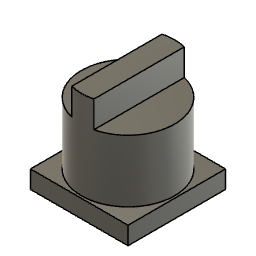
switch_knob (Autodesk Fusion 360 design; units mm, degrees)
Autodesk Fusion 360 part; units mm, degrees
sketch "Sketch1" plane through (0, 0, 0) normal (0, 1, 0) x (1, 0, 0)
  line L0 (5.5, 5.5) -> (-5.5, 5.5)
  line L1 (-5.5, 5.5) -> (-5.5, -5.5)
  line L2 (-5.5, -5.5) -> (5.5, -5.5)
  line L3 (5.5, -5.5) -> (5.5, 5.5)
  line L4 (5.5, 5.5) -> (-5.5, -5.5) construction
  line L5 (-5.5, 5.5) -> (5.5, -5.5) construction
  dimension "d1" = 11
  dimension "d2" = 11
  constraint horizontal L0
  constraint perpendicular L0 L1
  constraint parallel L0 L2
  constraint parallel L1 L3
  constraint coincident L4 origin
  constraint coincident L5 origin
  measures "d1" distance of L1.end L2.end
  measures "d2" distance of L0.end L1.end
extrude "Extrude1" add sketch "Sketch1" along normal blind 2
sketch "Sketch2" plane through (0, 2, 0) normal (0, 1, 0) x (-1, 0, 0)
  line L0 (-5.5, 5.5) -> (-5.5, -5.5)
  line L1 (-5.5, -5.5) -> (5.5, -5.5)
  line L2 (5.5, -5.5) -> (5.5, 5.5)
  line L3 (5.5, 5.5) -> (-5.5, 5.5)
  circle A0 centre (0, 0) radius 5.25
  dimension "d5" = 10.5
  constraint coincident A0.centre origin
  measures "d5" diameter of A0
extrude "Extrude2" add sketch "Sketch2" along normal blind 7 contours A0
sketch "Sketch3" plane through (0, 9, 0) normal (0, 1, 0) x (-1, 0, 0)
  circle A0 centre (0, 0) radius 5.25
  line L0 (1.25, 5.25) -> (-1.25, 5.25)
  line L1 (-1.25, 5.25) -> (-1.25, -5.25)
  line L2 (-1.25, -5.25) -> (1.25, -5.25)
  line L3 (1.25, -5.25) -> (1.25, 5.25)
  line L4 (1.25, 5.25) -> (-1.25, -5.25) construction
  line L5 (-1.25, 5.25) -> (1.25, -5.25) construction
  dimension "d8" = 2.5
  dimension "d9" = 10.5
  constraint horizontal L0
  constraint perpendicular L0 L1
  constraint parallel L0 L2
  constraint parallel L1 L3
  constraint coincident L4 A0.centre
  constraint coincident L5 A0.centre
  constraint coincident A0.centre origin
  measures "d8" distance of L1.end L2.end
  measures "d9" distance of L0.end L1.end
extrude "Extrude3" add sketch "Sketch3" along normal blind 3 contours A0 L1 L3
sketch "Sketch4" plane through (0, 0, 0) normal (0, -1, 0) x (1, 0, 0)
  line L0 (5.5, -5.5) -> (5.5, 5.5)
  line L1 (5.5, 5.5) -> (-5.5, 5.5)
  line L2 (-5.5, 5.5) -> (-5.5, -5.5)
  line L3 (-5.5, -5.5) -> (5.5, -5.5)
  line L4 (1.05, 1.55) -> (-1.05, 1.55)
  line L5 (-1.05, 1.55) -> (-1.05, -1.55)
  line L6 (-1.05, -1.55) -> (1.05, -1.55)
  line L7 (1.05, -1.55) -> (1.05, 1.55)
  line L8 (1.05, 1.55) -> (-1.05, -1.55) construction
  line L9 (-1.05, 1.55) -> (1.05, -1.55) construction
  dimension "d12" = 2.1
  dimension "d13" = 3.1
  constraint horizontal L4
  constraint perpendicular L4 L5
  constraint parallel L4 L6
  constraint parallel L5 L7
  constraint coincident L8 origin
  constraint coincident L9 origin
  measures "d12" distance of L5.end L6.end
  measures "d13" distance of L4.end L5.end
extrude "Extrude4" cut sketch "Sketch4" against normal blind 3 contours L4 L5 L6 L7
